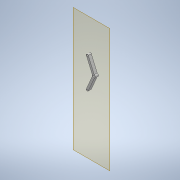
# Autodesk Inventor part: Шаблон
Saved by Autodesk Inventor 2020 (Build 240168000, 168)
## iProperties
Created: 2021-05-10
Part Number: Шаблон
Material: Типовые
Document SubType Name: Modeling
Designer: I_Love_U_Bogdan
Density: 1 g/cm^3
Appearance: По умолчанию
Author: I_Love_U_Bogdan
Autodesk Inventor part; units mm, degrees
ref_plane "YZ Plane" through (0, 0, 0) normal (1, 0, 0) x (0, 1, 0)
ref_plane "XZ Plane" through (0, 0, 0) normal (0, 1, 0) x (-1, 0, 0)
ref_plane "XY Plane" through (0, 0, 0) normal (0, 0, 1) x (1, 0, 0)
ref_plane "РабПлоскость1" through (0, 0, 0) normal (0, 0, 1) x (1, 0, 0)
sketch "Эскиз1" plane through (0, 0, 0) normal (0, 0, 1) x (1, 0, 0)
  circle A0 centre (43.2836, -60.3339) radius 1.5 projected
  circle A1 centre (43.2836, -130.3339) radius 1.5 projected
  circle A2 centre (43.2836, -60.3339) radius 1.6
  circle A3 centre (43.2836, -130.3339) radius 1.6
  line L0 (43.2836, -60.3339) -> (43.2836, -130.3339)
  line L1 (43.2836, -95.3339) -> (58.2836, -95.3339)
  circle A4 centre (58.2836, -95.3339) radius 2
  circle A5 centre (58.2836, -95.3339) radius 4
  line L2 (58.2836, -95.3339) -> (43.2836, -60.3339) construction
  line L3 (60.5815, -94.3491) -> (45.5815, -59.3491)
  line L4 (40.9858, -61.3187) -> (55.9858, -96.3187)
  arc A6 (55.9858, -96.3187) -> (60.5815, -94.3491) centre (58.2836, -95.3339) ccw
  arc A7 (45.5815, -59.3491) -> (40.9858, -61.3187) centre (43.2836, -60.3339) ccw
  line L5 (58.2836, -95.3339) -> (43.2836, -130.3339) construction
  line L6 (55.9858, -94.3491) -> (40.9858, -129.3491)
  line L7 (45.5815, -131.3187) -> (60.5815, -96.3187)
  arc A8 (60.5815, -96.3187) -> (55.9858, -94.3491) centre (58.2836, -95.3339) ccw
  arc A9 (40.9858, -129.3491) -> (45.5815, -131.3187) centre (43.2836, -130.3339) ccw
  point P0 (0, 0)
  point P1 (50.7836, -77.8339)
  point P2 (50.7836, -112.8339)
  point P3 (59.3515, -99.1887)
  point P4 (59.3515, -91.4791)
  point P5 (54.7558, -93.4487)
  point P6 (54.7558, -97.2191)
  dimension "d0" = 3.2
  dimension "d1" = 3.2
  dimension "d2" = 15
  dimension "d3" = 4
  dimension "d4" = 8
  dimension "d5" = 5
  dimension "d6" = 5
  constraints: 20 end point, 8 centre point, 8 point on circle, 8 tangent, 4 coincident, 3 midpoint, 2 parallel, 1 horizontal, 1 vertical
  measures "d0" diameter of A2
  measures "d1" diameter of A3
  measures "d2" distance of L1.start L1.end
  measures "d3" diameter of A4
  measures "d4" diameter of A5
  measures "d5" diameter of A7
  measures "d6" diameter of A9
extrude "Выдавливание1" add sketch "Эскиз1" along normal blind 7 contours L4 A7 L3 A5 | L4 L1 A5 | A5 L3 A8 L6 L4 | L6 A5 L7 A9 | L1 L6 A5 | A5 L7 A6 L3 | L6 A8 A6 L4 | L4 A6 L7 A5 L6
